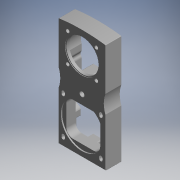
# Autodesk Inventor part: 1465008 EAMM-U-145-D100-140A-348S---(UT)
Saved by Autodesk Inventor 2017.3 (Build 213256000, 256)
## iProperties
Part Number: 1465008 EAMM-U-145-D100-140A-348S---(UT)
Material: Generic
Catalog Web Link: www.cadenas.de
Description: EAMM-U---(UT)-parallel kit
Vendor: FESTO
Document SubType Name: Modeling
Designer: partserver
Manufacturer: FESTO
Mass: 1054.09 g
Surface Area: 1717.35 cm^2
Volume: 1054.09 cm^3
Density: 1 g/cm^3
Appearance: PSOLRGB-192-192-192
Category: PARTsolutions
Company: FESTO
Title: 1465008 EAMM-U-145-D100-140A-348S---(UT)
Author: Cadenas PARTsolutions
Comments: parallel kit
PSOL_IDENT_0: {$CADENAS_DATA\23d-libs\festo\parts\e\eamm\parts\eamm_u_ut.prj},228 {VTYP=3D},{NB=1465008 EAMM-U-145
PSOL_IDENT_1: -D100-140A-348S---(UT)},{LINA=1465008 EAMM-U-145-D100-140A-348S---(UT)},{NN=EAMM-U---(UT)},{DATE=08.
PSOL_IDENT_2: 03.2021 13:38:17},{GEOMDATE=08.03.2021 13:37:58},{VERSION=},{LINEID=700},{WBVAR=},{WBNUMERIC=}  {NB=
PSOL_IDENT_3: 1465008 EAMM-U-145-D100-140A-348S---(UT)},{LINA=1465008 EAMM-U-145-D100-140A-348S---(UT)},{KT=DUMMY}
PSOL_IDENT_4: ,{TNR=1465008},{TYP=EAMM-U-145-D100-140A-348S},{VERS=5S},{VERS2=140A},{VERS3=D100},{W1=89.000},{W2=8
PSOL_IDENT_5: 9.000},{H0=188.000},{H5=70.000},{H7=348.000},{H8=94.000},{H10=193.000},{H12=345.000},{L1=49.500},{L4=
PSOL_IDENT_6: 12.500},{L4A=0.000},{L5=0.000},{L6=0.000},{D4=105.000},{T2=3.800},{T3=0.000},{T4=1.500},{SAX=58.3363
PSOL_IDENT_7: 09},{SAY=58.336309},{H1=45.000},{ANZ=4},{DV3=0.000},{DV2=0.000},{DV4=0.000},{DV5=0.000},{DV6=0.000},
PSOL_IDENT_8: {TV2=0.000},{LV2=0.000},{DM1=0.000},{DM2=0.000},{TM2=0.000},{LM1=0.000},{DM3=0.000},{DM4=0.000},{LM4=
PSOL_IDENT_9: 0.000},{RM4=0.000},{DM5=0.000},{LE1=0.000},{TV4=0.000},{TM3=0.000},{VR=0},{VRS=0},{T1=45.000}
NB: 1465008 EAMM-U-145-D100-140A-348S---(UT)
NN: EAMM-U---(UT)
NT: parallel kit
NBSYN: $TNR. $TYP.---(UT)
LINA: 1465008 EAMM-U-145-D100-140A-348S---(UT)
CATALOG: Festo
TNR: 1465008
TYP: EAMM-U-145-D100-140A-348S
VERS: 5S
VERS2: 140A
VERS3: D100
W1: 89
W2: 89
H0: 188
H5: 70
H7: 348
H8: 94
H10: 193
H12: 345
L1: 49.5
L4: 12.5
L4A: 0
L5: 0
L6: 0
D4: 105
T2: 3.8
T3: 0
T4: 1.5
H1: 45
ANZ: 4
VR: 0
VRS: 0
SUPPLIER: FESTO
ARTICLENO: 1465008 EAMM-U-145-D100-140A-348S---(UT)
BOMINFO: 1465008 EAMM-U-145-D100-140A-348S---(UT)
CREATOR: CADENAS GmbH
Autodesk Inventor part; units mm, degrees
sketch "Sketch_1" plane through (0, 0, 0) normal (0, 1, 0) x (-1, 0, 0)
  line L0 (72.5, -155.6275) -> (72.5, -6.3371)
  arc A0 (72.5, -6.3371) -> (71.2034, -4.8509) centre (71, -6.3371) ccw
  arc A1 (71.2034, -4.8509) -> (-71.2034, -4.8509) centre (0, -525) ccw
  arc A2 (-71.2034, -4.8509) -> (-72.5, -6.3371) centre (-71, -6.3371) ccw
  line L1 (-72.5, -6.3371) -> (-72.5, -155.6275)
  arc A3 (-72.5, -155.6275) -> (-72.3193, -156.653) centre (-69.5, -155.6275) ccw
  arc A4 (-72.3193, -211.347) -> (-72.3193, -156.653) centre (-147.5, -184) ccw
  arc A5 (-72.3193, -211.347) -> (-72.5, -212.3725) centre (-69.5, -212.3725) ccw
  line L2 (-72.5, -212.3725) -> (-72.5, -341.6629)
  arc A6 (-72.5, -341.6629) -> (-71.2034, -343.1491) centre (-71, -341.6629) ccw
  arc A7 (-71.2034, -343.1491) -> (71.2034, -343.1491) centre (0, 177) ccw
  arc A8 (71.2034, -343.1491) -> (72.5, -341.6629) centre (71, -341.6629) ccw
  line L3 (72.5, -341.6629) -> (72.5, -212.3725)
  arc A9 (72.5, -212.3725) -> (72.3193, -211.347) centre (69.5, -212.3725) ccw
  arc A10 (72.3193, -156.653) -> (72.3193, -211.347) centre (147.5, -184) ccw
  arc A11 (72.3193, -156.653) -> (72.5, -155.6275) centre (69.5, -155.6275) ccw
  constraints: 24 point on circle, 12 centre point, 8 end point
extrude "Extrusion1" add sketch "Sketch_1" along normal blind 49.5
sketch "Sketch_2" plane through (0, 0, 0) normal (1, 0, 0) x (0, 1, 0)
  line L0 (7.5, 0) -> (0, 0)
  line L1 (0, 0) -> (0, -7.5)
  line L2 (0, -7.5) -> (7.5, 0)
  constraints: 6 end point
extrude "Extrusion2" cut sketch "Sketch_2" along normal mid plane 145
sketch "Sketch_52" plane through (0, 49.5, 0) normal (0, 1, 0) x (1, 0, 0)
  line L0 (-71, 155.8931) -> (-71, 7.6474)
  arc A0 (-71, 7.6474) -> (-69.6997, 6.1607) centre (-69.5, 7.6474) ccw
  arc A1 (-69.6997, 6.1607) -> (69.6997, 6.1607) centre (0, 525) ccw
  arc A2 (69.6997, 6.1607) -> (71, 7.6474) centre (69.5, 7.6474) ccw
  line L1 (71, 7.6474) -> (71, 155.8931)
  arc A3 (71, 212.1069) -> (71, 155.8931) centre (147.5, 184) ccw
  line L2 (71, 212.1069) -> (71, 340.3526)
  arc A4 (71, 340.3526) -> (69.6997, 341.8393) centre (69.5, 340.3526) ccw
  arc A5 (69.6997, 341.8393) -> (-69.6997, 341.8393) centre (0, -177) ccw
  arc A6 (-69.6997, 341.8393) -> (-71, 340.3526) centre (-69.5, 340.3526) ccw
  line L3 (-71, 340.3526) -> (-71, 212.1069)
  arc A7 (-71, 155.8931) -> (-71, 212.1069) centre (-147.5, 184) ccw
  constraints: 16 point on circle, 8 centre point, 8 end point
extrude "Extrusion3" cut sketch "Sketch_52" against normal blind 0.75
sketch "Sketch4" plane through (0, 48.75, 0) normal (0, 1, 0) x (1, 0, 0)
  point P0 (8, 215)
hole "Hole1" at (8, 48.75, -215) direction (0, -1, 0) diameter 6.647 depth 18 tip angle 120 countersink diameter 8 countersink angle 90 thread size "M8x1.25" class "6H" standard "ISO Metric profile"
sketch "Sketch5" plane through (0, 48.75, 0) normal (0, 1, 0) x (1, 0, 0)
  point P0 (8, 153)
hole "Hole2" at (8, 48.75, -153) direction (0, -1, 0) diameter 6.647 depth 18 tip angle 120 countersink diameter 8 countersink angle 90 thread size "M8x1.25" class "6H" standard "ISO Metric profile"
sketch "Sketch6" plane through (0, 48.75, 0) normal (0, 1, 0) x (1, 0, 0)
  point P0 (-8, 215)
hole "Hole3" at (-8, 48.75, -215) direction (0, -1, 0) diameter 6.647 depth 18 tip angle 120 countersink diameter 8 countersink angle 90 thread size "M8x1.25" class "6H" standard "ISO Metric profile"
sketch "Sketch7" plane through (0, 48.75, 0) normal (0, 1, 0) x (1, 0, 0)
  point P0 (-8, 153)
hole "Hole4" at (-8, 48.75, -153) direction (0, -1, 0) diameter 6.647 depth 18 tip angle 120 countersink diameter 8 countersink angle 90 thread size "M8x1.25" class "6H" standard "ISO Metric profile"
sketch "Sketch8" plane through (0, 48.75, 0) normal (0, 1, 0) x (1, 0, 0)
  point P0 (-57.5, 313)
hole "Hole5" at (-57.5, 48.75, -313) direction (0, -1, 0) diameter 6.647 depth 15 tip angle 120 countersink diameter 8 countersink angle 90 thread size "M8x1.25" class "6H" standard "ISO Metric profile"
sketch "Sketch9" plane through (0, 48.75, 0) normal (0, 1, 0) x (1, 0, 0)
  point P0 (-57.5, 208)
hole "Hole6" at (-57.5, 48.75, -208) direction (0, -1, 0) diameter 6.647 depth 15 tip angle 120 countersink diameter 8 countersink angle 90 thread size "M8x1.25" class "6H" standard "ISO Metric profile"
sketch "Sketch10" plane through (0, 48.75, 0) normal (0, 1, 0) x (1, 0, 0)
  point P0 (57.5, 313)
hole "Hole7" at (57.5, 48.75, -313) direction (0, -1, 0) diameter 6.647 depth 15 tip angle 120 countersink diameter 8 countersink angle 90 thread size "M8x1.25" class "6H" standard "ISO Metric profile"
sketch "Sketch11" plane through (0, 48.75, 0) normal (0, 1, 0) x (1, 0, 0)
  point P0 (57.5, 208)
hole "Hole8" at (57.5, 48.75, -208) direction (0, -1, 0) diameter 6.647 depth 15 tip angle 120 countersink diameter 8 countersink angle 90 thread size "M8x1.25" class "6H" standard "ISO Metric profile"
sketch "Sketch12" plane through (0, 48.75, 0) normal (0, 1, 0) x (1, 0, 0)
  point P0 (0, 15)
hole "Hole9" at (0, 48.75, -15) direction (0, -1, 0) diameter 6.647 depth 15 tip angle 120 countersink diameter 8 countersink angle 90 thread size "M8x1.25" class "6H" standard "ISO Metric profile"
sketch "Sketch_23" plane through (0, 0, 0) normal (1, 0, 0) x (0, 1, 0)
  line L0 (0, -278) -> (49.5, -278)
  line L1 (49.5, -278) -> (49.5, -303)
  line L2 (49.5, -303) -> (2.1, -303)
  line L3 (2.1, -303) -> (1.5, -303.6)
  line L4 (1.5, -303.6) -> (1.5, -330.5)
  line L5 (1.5, -330.5) -> (0.2, -330.5)
  line L6 (0.2, -330.5) -> (0, -330.7)
  line L7 (0, -330.7) -> (0, -278)
  line L8 (0, -278) -> (49.5, -278)
  constraints: 18 end point
revolve "Revolution1" cut sketch "Sketch_23" angle 360 about axis through (0, 0, -278) along (0, -1, 0)
sketch "Sketch_45" plane through (0, 0, 0) normal (1, 0, 0) x (0, 1, 0)
  line L0 (0, -278) -> (49.5, -278)
  line L1 (49.5, -278) -> (49.5, -318)
  line L2 (49.5, -318) -> (1.5, -318)
  line L3 (1.5, -318) -> (1.5, -330.5)
  line L4 (1.5, -330.5) -> (0, -330.5)
  line L5 (0, -330.5) -> (0, -278)
  line L6 (0, -278) -> (49.5, -278)
  constraints: 14 end point
revolve "Revolution2" cut sketch "Sketch_45" angle 360 about axis through (0, 0, -278) along (0, -1, 0)
sketch "Sketch_47" plane through (0, 0, 0) normal (1, 0, 0) x (0, 1, 0)
  line L0 (0, -278) -> (49.5, -278)
  line L1 (49.5, -278) -> (49.5, -328)
  line L2 (49.5, -328) -> (1.5, -328)
  line L3 (1.5, -328) -> (1.5, -330.5)
  line L4 (1.5, -330.5) -> (0, -330.5)
  line L5 (0, -330.5) -> (0, -278)
  line L6 (0, -278) -> (49.5, -278)
  constraints: 14 end point
revolve "Revolution3" cut sketch "Sketch_47" angle 360 about axis through (0, 0, -278) along (0, -1, 0)
sketch "Sketch_22" plane through (44.5, 0, 0) normal (1, 0, 0) x (0, 0, -1)
  line L0 (233.5, 0) -> (233.5, 49.5)
  line L1 (233.5, 49.5) -> (242.5, 49.5)
  line L2 (242.5, 49.5) -> (242.5, 4.5)
  line L3 (242.5, 4.5) -> (239, 4.5)
  line L4 (239, 4.5) -> (239, 0)
  line L5 (239, 0) -> (233.5, 0)
  line L6 (233.5, 0) -> (233.5, 49.5)
  constraints: 14 end point
revolve "Revolution4" cut sketch "Sketch_22" angle 360 about axis through (44.5, 0, -233.5) along (0, -1, 0)
sketch "Sketch_30" plane through (44.5, 0, 0) normal (1, 0, 0) x (0, 0, -1)
  line L0 (322.5, 0) -> (322.5, 49.5)
  line L1 (322.5, 49.5) -> (331.5, 49.5)
  line L2 (331.5, 49.5) -> (331.5, 4.5)
  line L3 (331.5, 4.5) -> (328, 4.5)
  line L4 (328, 4.5) -> (328, 0)
  line L5 (328, 0) -> (322.5, 0)
  line L6 (322.5, 0) -> (322.5, 49.5)
  constraints: 14 end point
revolve "Revolution5" cut sketch "Sketch_30" angle 360 about axis through (44.5, 0, -322.5) along (0, -1, 0)
sketch "Sketch_35" plane through (-44.5, 0, 0) normal (1, 0, 0) x (0, 0, -1)
  line L0 (233.5, 0) -> (233.5, 49.5)
  line L1 (233.5, 49.5) -> (242.5, 49.5)
  line L2 (242.5, 49.5) -> (242.5, 4.5)
  line L3 (242.5, 4.5) -> (239, 4.5)
  line L4 (239, 4.5) -> (239, 0)
  line L5 (239, 0) -> (233.5, 0)
  line L6 (233.5, 0) -> (233.5, 49.5)
  constraints: 14 end point
revolve "Revolution6" cut sketch "Sketch_35" angle 360 about axis through (-44.5, 0, -233.5) along (0, -1, 0)
sketch "Sketch_40" plane through (-44.5, 0, 0) normal (1, 0, 0) x (0, 0, -1)
  line L0 (322.5, 0) -> (322.5, 49.5)
  line L1 (322.5, 49.5) -> (331.5, 49.5)
  line L2 (331.5, 49.5) -> (331.5, 4.5)
  line L3 (331.5, 4.5) -> (328, 4.5)
  line L4 (328, 4.5) -> (328, 0)
  line L5 (328, 0) -> (322.5, 0)
  line L6 (322.5, 0) -> (322.5, 49.5)
  constraints: 14 end point
revolve "Revolution7" cut sketch "Sketch_40" angle 360 about axis through (-44.5, 0, -322.5) along (0, -1, 0)
sketch "Sketch_31" plane through (0, 49.5, 0) normal (0, 1, 0) x (1, 0, 0)
  arc A0 (53.0863, 29.1637) -> (63.5863, 29.1637) centre (58.3363, 29.1637) ccw
  line L0 (63.5863, 29.1637) -> (63.5863, 34.1637)
  arc A1 (63.5863, 34.1637) -> (53.0863, 34.1637) centre (58.3363, 34.1637) ccw
  line L1 (53.0863, 34.1637) -> (53.0863, 29.1637)
  constraints: 4 end point, 4 point on circle, 2 centre point
extrude "Extrusion4" cut sketch "Sketch_31" against normal blind 49.5
sketch "Sketch_32" plane through (0, 49.5, 0) normal (0, 1, 0) x (1, 0, 0)
  arc A0 (53.0863, 145.8363) -> (63.5863, 145.8363) centre (58.3363, 145.8363) ccw
  line L0 (63.5863, 145.8363) -> (63.5863, 150.8363)
  arc A1 (63.5863, 150.8363) -> (53.0863, 150.8363) centre (58.3363, 150.8363) ccw
  line L1 (53.0863, 150.8363) -> (53.0863, 145.8363)
  constraints: 4 end point, 4 point on circle, 2 centre point
extrude "Extrusion5" cut sketch "Sketch_32" against normal blind 49.5
sketch "Sketch_33" plane through (0, 49.5, 0) normal (0, 1, 0) x (1, 0, 0)
  arc A0 (-63.5863, 145.8363) -> (-53.0863, 145.8363) centre (-58.3363, 145.8363) ccw
  line L0 (-53.0863, 145.8363) -> (-53.0863, 150.8363)
  arc A1 (-53.0863, 150.8363) -> (-63.5863, 150.8363) centre (-58.3363, 150.8363) ccw
  line L1 (-63.5863, 150.8363) -> (-63.5863, 145.8363)
  constraints: 4 end point, 4 point on circle, 2 centre point
extrude "Extrusion6" cut sketch "Sketch_33" against normal blind 49.5
sketch "Sketch_34" plane through (0, 49.5, 0) normal (0, 1, 0) x (1, 0, 0)
  arc A0 (-63.5863, 29.1637) -> (-53.0863, 29.1637) centre (-58.3363, 29.1637) ccw
  line L0 (-53.0863, 29.1637) -> (-53.0863, 34.1637)
  arc A1 (-53.0863, 34.1637) -> (-63.5863, 34.1637) centre (-58.3363, 34.1637) ccw
  line L1 (-63.5863, 34.1637) -> (-63.5863, 29.1637)
  constraints: 4 end point, 4 point on circle, 2 centre point
extrude "Extrusion7" cut sketch "Sketch_34" against normal blind 49.5
sketch "Sketch_29" plane through (0, 0, 0) normal (0, 1, 0) x (-1, 0, 0)
  arc A0 (65.25, -87.5) -> (-65.25, -87.5) centre (0, -87.5) ccw
  line L0 (-65.25, -87.5) -> (-65.25, -92.5)
  arc A1 (-65.25, -92.5) -> (65.25, -92.5) centre (0, -92.5) ccw
  line L1 (65.25, -92.5) -> (65.25, -87.5)
  constraints: 4 end point, 4 point on circle, 2 centre point
extrude "Extrusion8" cut sketch "Sketch_29" along normal blind 3.8
sketch "Sketch_4" plane through (0, 49.5, 0) normal (0, 1, 0) x (1, 0, 0)
  arc A0 (-50, 106.0078) -> (50, 106.0078) centre (0, 90) ccw
  line L0 (50, 106.0078) -> (50, 261.5303)
  arc A1 (50.1351, 262.4206) -> (50, 261.5303) centre (53, 261.5303) ccw
  arc A2 (50.1351, 262.4206) -> (-50.1351, 262.4206) centre (0, 278) ccw
  arc A3 (-50, 261.5303) -> (-50.1351, 262.4206) centre (-53, 261.5303) ccw
  line L1 (-50, 261.5303) -> (-50, 106.0078)
  line L2 (-16, 222.5) -> (-16, 145.5)
  arc A4 (-16, 145.5) -> (-13, 142.5) centre (-13, 145.5) ccw
  line L3 (-13, 142.5) -> (13, 142.5)
  arc A5 (13, 142.5) -> (16, 145.5) centre (13, 145.5) ccw
  line L4 (16, 145.5) -> (16, 222.5)
  arc A6 (16, 222.5) -> (13, 225.5) centre (13, 222.5) ccw
  line L5 (13, 225.5) -> (-13, 225.5)
  arc A7 (-13, 225.5) -> (-16, 222.5) centre (-13, 222.5) ccw
  constraints: 16 point on circle, 12 end point, 8 centre point
extrude "Extrusion9" cut sketch "Sketch_4" against normal blind 39
sketch "Sketch_49" plane through (0, 49.5, 0) normal (0, 1, 0) x (1, 0, 0)
  arc A0 (-52, 238.4749) -> (-52, 228.5251) centre (-44.5, 233.5) ccw
  arc A1 (-50, 221.8918) -> (-52, 228.5251) centre (-62, 221.8918) ccw
  line L0 (-50, 221.8918) -> (-50, 106.0078)
  arc A2 (-50, 106.0078) -> (50, 106.0078) centre (0, 90) ccw
  line L1 (50, 106.0078) -> (50, 221.8918)
  arc A3 (52, 228.5251) -> (50, 221.8918) centre (62, 221.8918) ccw
  arc A4 (52, 228.5251) -> (52, 238.4749) centre (44.5, 233.5) ccw
  arc A5 (50, 245.1082) -> (52, 238.4749) centre (62, 245.1082) ccw
  line L2 (50, 245.1082) -> (50, 261.9922)
  arc A6 (50, 261.9922) -> (-50, 261.9922) centre (0, 278) ccw
  line L3 (-50, 261.9922) -> (-50, 245.1082)
  arc A7 (-52, 238.4749) -> (-50, 245.1082) centre (-62, 245.1082) ccw
  line L4 (-16, 222.5) -> (-16, 145.5)
  arc A8 (-16, 145.5) -> (-13, 142.5) centre (-13, 145.5) ccw
  line L5 (-13, 142.5) -> (13, 142.5)
  arc A9 (13, 142.5) -> (16, 145.5) centre (13, 145.5) ccw
  line L6 (16, 145.5) -> (16, 222.5)
  arc A10 (16, 222.5) -> (13, 225.5) centre (13, 222.5) ccw
  line L7 (13, 225.5) -> (-13, 225.5)
  arc A11 (-13, 225.5) -> (-16, 222.5) centre (-13, 222.5) ccw
  constraints: 24 point on circle, 16 end point, 12 centre point
extrude "Extrusion10" cut sketch "Sketch_49" against normal blind 39
sketch "Sketch_53" plane through (0, 49.5, 0) normal (0, 1, 0) x (1, 0, 0)
  arc A0 (-66.8363, 103.2353) -> (-59.3527, 92.1177) centre (-54.8363, 103.2353) ccw
  arc A1 (-51.9864, 82.6744) -> (-59.3527, 92.1177) centre (-63.869, 81) ccw
  arc A2 (-51.9864, 82.6744) -> (-51.0606, 77.7907) centre (0, 90) ccw
  arc A3 (-58.7839, 63.6679) -> (-51.0606, 77.7907) centre (-62.7316, 75) ccw
  arc A4 (-58.7839, 63.6679) -> (-66.8363, 52.3358) centre (-54.8363, 52.3358) ccw
  line L0 (-66.8363, 52.3358) -> (-66.8363, 20.6637)
  arc A5 (-66.8363, 20.6637) -> (-54.8363, 8.6637) centre (-54.8363, 20.6637) ccw
  line L1 (-54.8363, 8.6637) -> (-28, 8.6637)
  arc A6 (-28, 8.6637) -> (-16, 20.6637) centre (-28, 20.6637) ccw
  line L2 (-16, 20.6637) -> (-16, 33.562)
  arc A7 (-10.0435, 38.4696) -> (-16, 33.562) centre (-11, 33.562) ccw
  arc A8 (-10.0435, 38.4696) -> (10.0435, 38.4696) centre (0, 90) ccw
  arc A9 (16, 33.562) -> (10.0435, 38.4696) centre (11, 33.562) ccw
  line L3 (16, 33.562) -> (16, 20.6637)
  arc A10 (16, 20.6637) -> (28, 8.6637) centre (28, 20.6637) ccw
  line L4 (28, 8.6637) -> (54.8363, 8.6637)
  arc A11 (54.8363, 8.6637) -> (66.8363, 20.6637) centre (54.8363, 20.6637) ccw
  line L5 (66.8363, 20.6637) -> (66.8363, 52.3358)
  arc A12 (66.8363, 52.3358) -> (58.7839, 63.6679) centre (54.8363, 52.3358) ccw
  arc A13 (51.0606, 77.7907) -> (58.7839, 63.6679) centre (62.7316, 75) ccw
  arc A14 (51.0606, 77.7907) -> (51.9864, 82.6744) centre (0, 90) ccw
  arc A15 (59.3527, 92.1177) -> (51.9864, 82.6744) centre (63.869, 81) ccw
  arc A16 (59.3527, 92.1177) -> (66.8363, 103.2353) centre (54.8363, 103.2353) ccw
  line L6 (66.8363, 103.2353) -> (66.8363, 159.3363)
  arc A17 (66.8363, 159.3363) -> (54.9519, 171.3358) centre (54.8363, 159.3363) ccw
  arc A18 (50, 176.3355) -> (54.9519, 171.3358) centre (55, 176.3355) ccw
  line L7 (50, 176.3355) -> (50, 261.9922)
  arc A19 (50, 261.9922) -> (-50, 261.9922) centre (0, 278) ccw
  line L8 (-50, 261.9922) -> (-50, 176.3355)
  arc A20 (-54.9519, 171.3358) -> (-50, 176.3355) centre (-55, 176.3355) ccw
  arc A21 (-54.9519, 171.3358) -> (-66.8363, 159.3363) centre (-54.8363, 159.3363) ccw
  line L9 (-66.8363, 159.3363) -> (-66.8363, 103.2353)
  line L10 (-16, 222.5) -> (-16, 145.5)
  arc A22 (-16, 145.5) -> (-13, 142.5) centre (-13, 145.5) ccw
  line L11 (-13, 142.5) -> (13, 142.5)
  arc A23 (13, 142.5) -> (16, 145.5) centre (13, 145.5) ccw
  line L12 (16, 145.5) -> (16, 222.5)
  arc A24 (16, 222.5) -> (13, 225.5) centre (13, 222.5) ccw
  line L13 (13, 225.5) -> (-13, 225.5)
  arc A25 (-13, 225.5) -> (-16, 222.5) centre (-13, 222.5) ccw
  constraints: 52 point on circle, 28 end point, 26 centre point
extrude "Extrusion11" cut sketch "Sketch_53" against normal blind 17
sketch "Sketch28" plane through (0, 48.75, 0) normal (0, 1, 0) x (1, 0, 0)
  point P0 (57.5, 78)
hole "Hole10" at (57.5, 48.75, -78) direction (0, -1, 0) diameter 6.647 depth 15 tip angle 120 countersink diameter 8 countersink angle 90 thread size "M8x1.25" class "6H" standard "ISO Metric profile"
sketch "Sketch29" plane through (0, 48.75, 0) normal (0, 1, 0) x (1, 0, 0)
  point P0 (-57.5, 78)
hole "Hole11" at (-57.5, 48.75, -78) direction (0, -1, 0) diameter 6.647 depth 15 tip angle 120 countersink diameter 8 countersink angle 90 thread size "M8x1.25" class "6H" standard "ISO Metric profile"
sketch "Sketch_5" plane through (0, 0, 0) normal (1, 0, 0) x (0, 1, 0)
  line L0 (0, -90) -> (49.5, -90)
  line L1 (49.5, -90) -> (49.5, -115)
  line L2 (49.5, -115) -> (0, -115)
  line L3 (0, -115) -> (0, -90)
  line L4 (0, -90) -> (49.5, -90)
  constraints: 10 end point
revolve "Revolution8" cut sketch "Sketch_5" angle 360 about axis through (0, 0, -90) along (0, -1, 0)
sketch "Sketch31" plane through (0, 0, 0) normal (0, -1, 0) x (1, 0, 0)
  point P0 (0, -175)
hole "Hole12" at (0, 0, -175) direction (0, 1, 0) diameter 15.3 depth 12
sketch "Sketch_57" plane through (0, 0, 0) normal (0, 1, 0) x (-1, 0, 0)
  arc A0 (52.5, -57.5) -> (32.5, -37.5) centre (32.5, -57.5) ccw
  line L0 (32.5, -37.5) -> (-32.5, -37.5)
  arc A1 (-32.5, -37.5) -> (-52.5, -57.5) centre (-32.5, -57.5) ccw
  line L1 (-52.5, -57.5) -> (-52.5, -122.5)
  arc A2 (-52.5, -122.5) -> (-32.5, -142.5) centre (-32.5, -122.5) ccw
  line L2 (-32.5, -142.5) -> (32.5, -142.5)
  arc A3 (32.5, -142.5) -> (52.5, -122.5) centre (32.5, -122.5) ccw
  line L3 (52.5, -122.5) -> (52.5, -57.5)
  constraints: 8 end point, 8 point on circle, 4 centre point
extrude "Extrusion12" cut sketch "Sketch_57" along normal blind 50
ref_plane "ANBAU_XY" through (0, 0, -278) normal (0, 1, 0) x (1, 0, 0)
ref_plane "ANBAU_YZ" through (0, 0, -278) normal (1, 0, 0) x (0, 0, -1)
ref_plane "ANBAU_ZX" through (0, 0, -278) normal (0, 0, -1) x (0, 1, 0)
ref_plane "AS_1_XY" through (44.5, 4.5, -233.5) normal (0, 1, 0) x (1, 0, 0)
ref_plane "AS_1_YZ" through (44.5, 4.5, -233.5) normal (1, 0, 0) x (0, 0, -1)
ref_plane "AS_1_ZX" through (44.5, 4.5, -233.5) normal (0, 0, -1) x (0, 1, 0)
ref_plane "AS_2_XY" through (44.5, 4.5, -322.5) normal (0, 1, 0) x (1, 0, 0)
ref_plane "AS_2_YZ" through (44.5, 4.5, -322.5) normal (1, 0, 0) x (0, 0, -1)
ref_plane "AS_2_ZX" through (44.5, 4.5, -322.5) normal (0, 0, -1) x (0, 1, 0)
ref_plane "AS_3_XY" through (-44.5, 4.5, -233.5) normal (0, 1, 0) x (1, 0, 0)
ref_plane "AS_3_YZ" through (-44.5, 4.5, -233.5) normal (1, 0, 0) x (0, 0, -1)
ref_plane "AS_3_ZX" through (-44.5, 4.5, -233.5) normal (0, 0, -1) x (0, 1, 0)
ref_plane "AS_4_XY" through (-44.5, 4.5, -322.5) normal (0, 1, 0) x (1, 0, 0)
ref_plane "AS_4_YZ" through (-44.5, 4.5, -322.5) normal (1, 0, 0) x (0, 0, -1)
ref_plane "AS_4_ZX" through (-44.5, 4.5, -322.5) normal (0, 0, -1) x (0, 1, 0)
ref_plane "DM_XY" through (0, 0, -90) normal (0, 1, 0) x (1, 0, 0)
ref_plane "DM_YZ" through (0, 0, -90) normal (1, 0, 0) x (0, 0, -1)
ref_plane "DM_ZX" through (0, 0, -90) normal (0, 0, -1) x (0, 1, 0)
ref_plane "MS_1_XY" through (58.3363, -12.5, -31.6637) normal (0, 1, 0) x (1, 0, 0)
ref_plane "MS_1_YZ" through (58.3363, -12.5, -31.6637) normal (1, 0, 0) x (0, 0, -1)
ref_plane "MS_1_ZX" through (58.3363, -12.5, -31.6637) normal (0, 0, -1) x (0, 1, 0)
ref_plane "MS_2_XY" through (58.3363, -12.5, -148.3363) normal (0, 1, 0) x (1, 0, 0)
ref_plane "MS_2_YZ" through (58.3363, -12.5, -148.3363) normal (1, 0, 0) x (0, 0, -1)
ref_plane "MS_2_ZX" through (58.3363, -12.5, -148.3363) normal (0, 0, -1) x (0, 1, 0)
ref_plane "MS_3_XY" through (-58.3363, -12.5, -148.3363) normal (0, 1, 0) x (1, 0, 0)
ref_plane "MS_3_YZ" through (-58.3363, -12.5, -148.3363) normal (1, 0, 0) x (0, 0, -1)
ref_plane "MS_3_ZX" through (-58.3363, -12.5, -148.3363) normal (0, 0, -1) x (0, 1, 0)
ref_plane "MS_4_XY" through (-58.3363, -12.5, -31.6637) normal (0, 1, 0) x (1, 0, 0)
ref_plane "MS_4_YZ" through (-58.3363, -12.5, -31.6637) normal (1, 0, 0) x (0, 0, -1)
ref_plane "MS_4_ZX" through (-58.3363, -12.5, -31.6637) normal (0, 0, -1) x (0, 1, 0)
ref_plane "MS_A_1_XY" through (58.3363, 0, -31.6637) normal (0, 1, 0) x (1, 0, 0)
ref_plane "MS_A_1_YZ" through (58.3363, 0, -31.6637) normal (1, 0, 0) x (0, 0, -1)
ref_plane "MS_A_1_ZX" through (58.3363, 0, -31.6637) normal (0, 0, -1) x (0, 1, 0)
ref_plane "MS_A_2_XY" through (58.3363, 0, -148.3363) normal (0, 1, 0) x (1, 0, 0)
ref_plane "MS_A_2_YZ" through (58.3363, 0, -148.3363) normal (1, 0, 0) x (0, 0, -1)
ref_plane "MS_A_2_ZX" through (58.3363, 0, -148.3363) normal (0, 0, -1) x (0, 1, 0)
ref_plane "MS_A_3_XY" through (-58.3363, 0, -148.3363) normal (0, 1, 0) x (1, 0, 0)
ref_plane "MS_A_3_YZ" through (-58.3363, 0, -148.3363) normal (1, 0, 0) x (0, 0, -1)
ref_plane "MS_A_3_ZX" through (-58.3363, 0, -148.3363) normal (0, 0, -1) x (0, 1, 0)
ref_plane "MS_A_4_XY" through (-58.3363, 0, -31.6637) normal (0, 1, 0) x (1, 0, 0)
ref_plane "MS_A_4_YZ" through (-58.3363, 0, -31.6637) normal (1, 0, 0) x (0, 0, -1)
ref_plane "MS_A_4_ZX" through (-58.3363, 0, -31.6637) normal (0, 0, -1) x (0, 1, 0)
ref_plane "OBERTEIL_XY" through (0, 49.5, -278) normal (0, 1, 0) x (1, 0, 0)
ref_plane "OBERTEIL_YZ" through (0, 49.5, -278) normal (1, 0, 0) x (0, 0, -1)
ref_plane "OBERTEIL_ZX" through (0, 49.5, -278) normal (0, 0, -1) x (0, 1, 0)
ref_plane "VM_1_XY" through (58.3363, 32.5, -31.6637) normal (0, 1, 0) x (1, 0, 0)
ref_plane "VM_1_YZ" through (58.3363, 32.5, -31.6637) normal (1, 0, 0) x (0, 0, -1)
ref_plane "VM_1_ZX" through (58.3363, 32.5, -31.6637) normal (0, 0, -1) x (0, 1, 0)
ref_plane "VM_2_XY" through (58.3363, 32.5, -148.3363) normal (0, 1, 0) x (1, 0, 0)
ref_plane "VM_2_YZ" through (58.3363, 32.5, -148.3363) normal (1, 0, 0) x (0, 0, -1)
ref_plane "VM_2_ZX" through (58.3363, 32.5, -148.3363) normal (0, 0, -1) x (0, 1, 0)
ref_plane "VM_3_XY" through (-58.3363, 32.5, -148.3363) normal (0, 1, 0) x (1, 0, 0)
ref_plane "VM_3_YZ" through (-58.3363, 32.5, -148.3363) normal (1, 0, 0) x (0, 0, -1)
ref_plane "VM_3_ZX" through (-58.3363, 32.5, -148.3363) normal (0, 0, -1) x (0, 1, 0)
ref_plane "VM_4_XY" through (-58.3363, 32.5, -31.6637) normal (0, 1, 0) x (1, 0, 0)
ref_plane "VM_4_YZ" through (-58.3363, 32.5, -31.6637) normal (1, 0, 0) x (0, 0, -1)
ref_plane "VM_4_ZX" through (-58.3363, 32.5, -31.6637) normal (0, 0, -1) x (0, 1, 0)
ref_plane "VS_XY" through (0, 0, -175) normal (0, 1, 0) x (1, 0, 0)
ref_plane "VS_YZ" through (0, 0, -175) normal (1, 0, 0) x (0, 0, -1)
ref_plane "VS_ZX" through (0, 0, -175) normal (0, 0, -1) x (0, 1, 0)
ref_plane "ZR_XY" through (0, 1.5, -278) normal (0, 1, 0) x (1, 0, 0)
ref_plane "ZR_YZ" through (0, 1.5, -278) normal (1, 0, 0) x (0, 0, -1)
ref_plane "ZR_ZX" through (0, 1.5, -278) normal (0, 0, -1) x (0, 1, 0)
body "Solid1"
